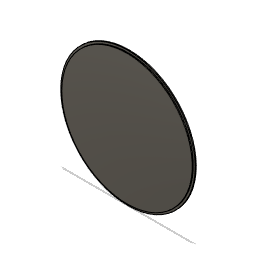
Uhr-Glas (Autodesk Fusion 360 design; units mm, degrees)
Autodesk Fusion 360 part; units mm, degrees
sketch "Skizze1" plane through (0, 0, 0) normal (0, 0, 1) x (1, 0, 0)
  circle A0 centre (0, 0) radius 103
  dimension "d1" = 206
  constraint coincident A0.centre origin
  measures "d1" diameter of A0
extrude "Extrusion1" add sketch "Skizze1" along normal blind 3
sketch "Skizze2" plane through (0, 0, 3) normal (0, 0, 1) x (1, 0, 0)
  circle A0 centre (0, 0) radius 103
  circle A1 centre (0, 0) radius 100
  dimension "d7" = 3
  constraint concentric A0 A1
  measures "d7" distance of A0 A1
extrude "Extrusion2" cut sketch "Skizze2" against normal blind 1.5
